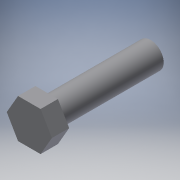
# Autodesk Inventor part: bolt
Saved by Autodesk Inventor 2016 (Build 200138000, 138)
## iProperties
Created: 2016-02-24
Part Number: bolt
Material: Steel, Galvanized
Document SubType Name: Modeling
Designer: gus
Density: 7.85 g/cm^3
Appearance: Galvanized
Author: gus
Autodesk Inventor part; units mm, degrees
ref_plane "YZ Plane" through (0, 0, 0) normal (1, 0, 0) x (0, 1, 0)
ref_plane "XZ Plane" through (0, 0, 0) normal (0, 1, 0) x (-1, 0, 0)
ref_plane "XY Plane" through (0, 0, 0) normal (0, 0, 1) x (1, 0, 0)
sketch "Sketch1" plane through (0, 0, 0) normal (0, 0, 1) x (1, 0, 0)
  line L0 (4.1244, 7.1437) -> (8.2489, 0)
  line L1 (8.2489, 0) -> (4.1244, -7.1438)
  line L2 (4.1244, -7.1438) -> (-4.1244, -7.1437)
  line L3 (-4.1244, -7.1437) -> (-8.2489, 0)
  line L4 (-8.2489, 0) -> (-4.1244, 7.1437)
  line L5 (-4.1244, 7.1437) -> (4.1244, 7.1437)
  point P0 (0, 0)
  point P1 (0, 0)
  dimension "d0" = 14.2875
  constraints: 12 end point, 1 coincident, 1 horizontal, 13 other
  measures "d0" distance between parallel lines of L2 L5
extrude "Extrusion1" add sketch "Sketch1" along normal blind 6.35
sketch "Sketch2" plane through (0, 0, 0) normal (0, 0, -1) x (-1, 0, 0)
  circle A0 centre (0, 0) radius 4.7625
  dimension "d3" = 9.525
  constraints: 1 centre point, 1 coincident
  measures "d3" diameter of A0
extrude "Extrusion2" add sketch "Sketch2" along normal blind 38.1
body "Solid1"
